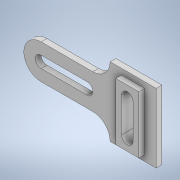
# Autodesk Inventor part: Ch3 Part 1
Saved by Autodesk Inventor 2020 (Build 240168000, 168)
## iProperties
Created: 2021-01-28
Part Number: Ch3 Part 1
Material: Generic
Document SubType Name: Modeling
Designer: austi
Density: 1 g/cm^3
Appearance: Default
Author: austi
Autodesk Inventor part; units mm, degrees
ref_plane "YZ Plane" through (0, 0, 0) normal (1, 0, 0) x (0, 1, 0)
ref_plane "XZ Plane" through (0, 0, 0) normal (0, 1, 0) x (-1, 0, 0)
ref_plane "XY Plane" through (0, 0, 0) normal (0, 0, 1) x (1, 0, 0)
sketch "Sketch1" plane through (0, 0, 0) normal (0, 0, 1) x (1, 0, 0)
  line L0 (0, -3.175) -> (25.4, -3.175)
  arc A0 (25.4, -3.175) -> (25.4, 3.175) centre (25.4, 0) ccw
  line L1 (25.4, 3.175) -> (0, 3.175)
  arc A1 (0, 3.175) -> (0, -3.175) centre (0, 0) ccw
  arc A2 (0, 9.525) -> (0, -9.525) centre (0, 0) ccw
  line L2 (0, 9.525) -> (28.575, 9.525)
  line L3 (0, -9.525) -> (28.575, -9.525)
  arc A3 (28.575, 9.525) -> (38.1, 19.05) centre (28.575, 19.05) ccw
  arc A4 (38.1, -19.05) -> (28.575, -9.525) centre (28.575, -19.05) ccw
  line L4 (38.1, -19.05) -> (63.5, -19.05)
  line L5 (38.1, 19.05) -> (63.5, 19.05)
  line L6 (44.45, 15.875) -> (57.15, 15.875)
  line L7 (53.975, 9.525) -> (53.975, -9.525)
  line L8 (47.625, -9.525) -> (47.625, 9.525)
  arc A5 (53.975, 9.525) -> (47.625, 9.525) centre (50.8, 9.525) ccw
  line L9 (44.45, 15.875) -> (44.45, -15.875)
  line L10 (44.45, -15.875) -> (57.15, -15.875)
  line L11 (57.15, 15.875) -> (57.15, -15.875)
  arc A6 (47.625, -9.525) -> (53.975, -9.525) centre (50.8, -9.525) ccw
  line L12 (-24.13, 0) -> (78.105, 0) projected
  line L13 (0, -26.67) -> (0, 26.67) projected
  line L14 (63.5, 19.05) -> (63.5, -19.05)
  point P0 (0, 0)
  point P1 (50.8, 12.7)
  point P2 (50.8, 15.875)
  point P3 (50.8, 19.05)
  point P4 (50.8, -19.05)
  point P5 (63.5, 0)
  point P6 (47.625, 0)
  point P7 (53.975, 0)
  point P8 (44.45, 0)
  point P9 (57.15, 0)
  dimension "d25" = 63.5
  dimension "d26" = 25.4
  dimension "d27" = 6.35
  dimension "d28" = 12.7
  dimension "d29" = 3.175
  dimension "d30" = 9.525
  dimension "d31" = 3.175
  dimension "d32" = 25.4
  dimension "d33" = 38.1
  dimension "d34" = 3.175
  dimension "d35" = 19.05
  dimension "d36" = 31.75
  constraints: 26 end point, 15 point on circle, 10 horizontal alignment, 8 midpoint, 8 vertical alignment, 7 centre point, 6 horizontal, 4 equal radius, 3 parallel, 3 tangent, 2 coincident, 2 line through centre, 2 perpendicular, 1 vertical, 1 other
  measures "d25" horizontal distance of L5.end point (0, 0)
  measures "d26" distance of L5.start L5.end
  measures "d27" horizontal distance of L5.end L6.end
  measures "d28" distance of L6.start L6.end
  measures "d29" radius of A6
  measures "d30" radius of A2
  measures "d31" radius of A1
  measures "d32" distance of A0.centre point (0, 0)
  measures "d33" distance of L4.end L5.end
  measures "d34" vertical distance of L5.end L6.end
  measures "d35" distance of A6.centre A5.centre
  measures "d36" distance of L6.end L10.end
extrude "Extrusion1" add sketch "Sketch1" along normal blind 3.175 contours L13 L12 A0 L0 | L13 A2 L12 A1 | L0 A0 L12 L9 L10 L11 L14 L4 A4 L3 L13 | A1 L12 L13 | L12 A2 L13 A1 | A1 L13 L12 | L13 L1 A0 L12 | A0 L1 L13 L2 A3 L5 L14 L12 L11 L6 L9
extrude "Extrusion2" add sketch "Sketch1" along normal blind 6.35 contours L12 L8 A6 L7 L11 L10 L9 | L9 L6 L11 L12 L7 A5 L8
sketch "Sketch2" plane through (0, 0, 3.175) normal (0, 0, 1) x (1, 0, 0)
  circle A0 centre (0, 0) radius 3.175
  line L0 (0, 3.175) -> (25.4, 3.175)
  circle A1 centre (25.4, 0) radius 3.175
  line L1 (0, -3.175) -> (25.4, -3.175)
  line L2 (-24.13, 0) -> (78.105, 0) projected
  dimension "d37" = 6.35
  dimension "d38" = 25.4
  constraints: 4 end point, 4 point on circle, 2 centre point, 2 tangent, 1 coincident, 1 equal radius, 1 horizontal, 1 horizontal alignment, 1 other
  measures "d37" diameter of A0
  measures "d38" distance of L0.start L0.end
extrude "Extrusion3" cut sketch "Sketch2" against normal through all
body "Solid1"
